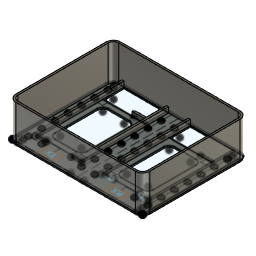
Pluto_Case_V2.8_lite (Autodesk Fusion 360 design; units mm, degrees)
Autodesk Fusion 360 part; units mm, degrees
sketch "base" plane through (0, 0, 0) normal (0, 0, 1) x (1, 0, 0)
  line L0 (10, 0) -> (235, 0)
  line L1 (245, 10) -> (245, 180)
  line L2 (235, 190) -> (10, 190)
  line L3 (0, 180) -> (0, 10)
  line L4 (0, 0) -> (10, 0) construction
  line L5 (0, 190) -> (10, 190) construction
  line L6 (10, 190) -> (10, 170) construction
  circle A0 centre (10, 170) radius 5
  line L7 (10, 170) -> (10, 145) construction
  line L8 (10, 145) -> (10, 120) construction
  line L9 (10, 120) -> (10, 95) construction
  line L10 (10, 95) -> (10, 70) construction
  line L11 (10, 70) -> (10, 45) construction
  line L12 (10, 45) -> (10, 20) construction
  circle A1 centre (10, 145) radius 5
  circle A2 centre (10, 120) radius 5
  circle A3 centre (10, 95) radius 5
  circle A4 centre (10, 70) radius 5
  circle A5 centre (10, 45) radius 5
  circle A6 centre (10, 20) radius 5
  line L13 (0, 190) -> (20, 190) construction
  line L14 (20, 190) -> (100, 190) construction
  line L15 (20, 190) -> (100, 190)
  line L16 (100, 190) -> (100, 150)
  line L17 (100, 150) -> (20, 150)
  line L18 (20, 160) -> (20, 190)
  line L19 (30, 150) -> (100, 150)
  line L20 (100, 150) -> (100, 30)
  line L21 (100, 30) -> (20, 30)
  line L22 (20, 30) -> (20, 150)
  line L23 (20, 150) -> (30, 150) construction
  line L24 (30, 150) -> (30, 140) construction
  line L25 (30, 140) -> (20, 140) construction
  line L26 (20, 140) -> (20, 150) construction
  line L27 (100, 30) -> (90, 30) construction
  line L28 (90, 30) -> (90, 40) construction
  line L29 (90, 40) -> (100, 40) construction
  line L30 (100, 40) -> (100, 30) construction
  line L31 (40, 140) -> (80, 140)
  line L32 (90, 130) -> (90, 50)
  line L33 (80, 40) -> (40, 40)
  line L34 (30, 50) -> (30, 130)
  line L35 (20, 190) -> (16, 190) construction
  line L36 (100, 190) -> (104, 190) construction
  line L37 (16, 190) -> (16, 30)
  line L38 (20, 26) -> (33, 26)
  line L39 (36, 29) -> (36, 30)
  line L40 (104, 190) -> (104, 30)
  line L41 (100, 26) -> (87, 26)
  line L42 (84, 29) -> (84, 30)
  line L43 (100, 190) -> (110, 190) construction
  line L44 (0, 0) -> (100, 0) construction
  line L45 (100, 0) -> (110, 0) construction
  line L46 (110, 190) -> (110, 170) construction
  line L47 (110, 170) -> (110, 145) construction
  line L48 (110, 145) -> (110, 120) construction
  line L49 (110, 120) -> (110, 95) construction
  line L50 (110, 95) -> (110, 70) construction
  line L51 (110, 70) -> (110, 45) construction
  line L52 (110, 45) -> (110, 20) construction
  circle A7 centre (110, 170) radius 5
  circle A8 centre (110, 145) radius 5
  circle A9 centre (110, 120) radius 5
  circle A10 centre (110, 95) radius 5
  circle A11 centre (110, 70) radius 5
  circle A12 centre (110, 45) radius 5
  circle A13 centre (110, 20) radius 5
  line L53 (0, 190) -> (122.5, 190) construction
  line L54 (0, 0) -> (122.5, 0) construction
  line L55 (122.5, 190) -> (122.5, 0) construction
  line L56 (10, 20) -> (35, 20) construction
  circle A14 centre (35, 20) radius 5
  arc A15 (40, 140) -> (30, 130) centre (40, 130) ccw
  arc A16 (90, 130) -> (80, 140) centre (80, 130) ccw
  arc A17 (80, 40) -> (90, 50) centre (80, 50) ccw
  arc A18 (30, 50) -> (40, 40) centre (40, 50) ccw
  arc A19 (16, 30) -> (20, 26) centre (20, 30) ccw
  arc A20 (100, 26) -> (104, 30) centre (100, 30) ccw
  circle A21 centre (135, 70) radius 5
  line L57 (155, 40) -> (145, 40) construction
  line L58 (235, 190) -> (235, 170) construction
  arc A22 (141, 30) -> (145, 26) centre (145, 30) ccw
  line L59 (141, 190) -> (141, 30)
  line L60 (145, 0) -> (135, 0) construction
  line L61 (145, 26) -> (158, 26)
  line L62 (145, 150) -> (145, 30)
  line L63 (225, 150) -> (215, 150) construction
  line L64 (225, 190) -> (229, 190) construction
  arc A23 (155, 50) -> (165, 40) centre (165, 50) ccw
  line L65 (209, 29) -> (209, 30)
  circle A24 centre (135, 45) radius 5
  line L66 (161, 29) -> (161, 30)
  line L67 (135, 45) -> (135, 20) construction
  circle A25 centre (135, 20) radius 5
  line L68 (245, 190) -> (225, 190) construction
  line L69 (245, 190) -> (235, 190) construction
  line L70 (155, 30) -> (155, 40) construction
  line L71 (235, 170) -> (235, 145) construction
  line L72 (145, 30) -> (155, 30) construction
  line L73 (145, 40) -> (145, 30) construction
  circle A26 centre (235, 170) radius 5
  line L74 (135, 70) -> (135, 45) construction
  line L75 (215, 150) -> (215, 140) construction
  line L76 (225, 190) -> (145, 190) construction
  circle A27 centre (235, 20) radius 5
  circle A28 centre (235, 145) radius 5
  arc A29 (225, 26) -> (229, 30) centre (225, 30) ccw
  arc A30 (205, 40) -> (215, 50) centre (205, 50) ccw
  circle A31 centre (235, 70) radius 5
  circle A32 centre (235, 120) radius 5
  line L77 (225, 150) -> (225, 190)
  circle A33 centre (210, 20) radius 5
  arc A34 (215, 130) -> (205, 140) centre (205, 130) ccw
  line L78 (215, 140) -> (225, 140) construction
  line L79 (235, 45) -> (235, 20) construction
  circle A35 centre (235, 45) radius 5
  line L80 (225, 140) -> (225, 150) construction
  line L81 (235, 145) -> (235, 120) construction
  line L82 (235, 120) -> (235, 95) construction
  line L83 (235, 20) -> (210, 20) construction
  line L84 (225, 26) -> (212, 26)
  line L85 (229, 190) -> (229, 30)
  line L86 (225, 30) -> (225, 150)
  line L87 (235, 70) -> (235, 45) construction
  line L88 (215, 50) -> (215, 130)
  circle A36 centre (235, 95) radius 5
  line L89 (235, 95) -> (235, 70) construction
  line L90 (205, 140) -> (165, 140)
  circle A37 centre (135, 95) radius 5
  line L91 (135, 190) -> (135, 170) construction
  line L92 (145, 190) -> (141, 190) construction
  line L93 (145, 30) -> (225, 30)
  line L94 (135, 120) -> (135, 95) construction
  line L95 (135, 145) -> (135, 120) construction
  circle A38 centre (135, 120) radius 5
  circle A39 centre (135, 145) radius 5
  circle A40 centre (135, 170) radius 5
  line L96 (145, 150) -> (225, 150)
  line L97 (225, 190) -> (145, 190)
  arc A41 (165, 140) -> (155, 130) centre (165, 130) ccw
  line L98 (225, 150) -> (155, 150)
  line L99 (135, 170) -> (135, 145) construction
  line L100 (145, 190) -> (145, 160)
  line L101 (245, 0) -> (145, 0) construction
  line L102 (135, 95) -> (135, 70) construction
  line L103 (245, 0) -> (235, 0) construction
  line L104 (155, 130) -> (155, 50)
  line L105 (145, 190) -> (135, 190) construction
  line L106 (165, 40) -> (205, 40)
  line L107 (100, 150) -> (75, 150)
  line L108 (79, 154) -> (100, 154)
  line L109 (100, 154) -> (100, 150)
  arc A42 (79, 154) -> (75, 150) centre (79, 150) ccw
  line L110 (225, 150) -> (200, 150)
  line L111 (204, 154) -> (225, 154)
  line L112 (225, 154) -> (225, 150)
  arc A43 (204, 154) -> (200, 150) centre (204, 150) ccw
  arc A44 (10, 190) -> (0, 180) centre (10, 180) ccw
  arc A45 (0, 10) -> (10, 0) centre (10, 10) ccw
  arc A46 (235, 0) -> (245, 10) centre (235, 10) ccw
  arc A47 (245, 180) -> (235, 190) centre (235, 180) ccw
  line L113 (235, 193.6) -> (10, 193.6)
  arc A48 (10, 193.6) -> (-3.6, 180) centre (10, 180) ccw
  line L114 (-3.6, 180) -> (-3.6, 10)
  arc A49 (-3.6, 10) -> (10, -3.6) centre (10, 10) ccw
  line L115 (10, -3.6) -> (235, -3.6)
  arc A50 (235, -3.6) -> (248.6, 10) centre (235, 10) ccw
  line L116 (248.6, 10) -> (248.6, 180)
  arc A51 (248.6, 180) -> (235, 193.6) centre (235, 180) ccw
  arc A52 (33, 26) -> (36, 29) centre (33, 29) ccw
  arc A53 (84, 29) -> (87, 26) centre (87, 29) ccw
  arc A54 (158, 26) -> (161, 29) centre (158, 29) ccw
  arc A55 (209, 29) -> (212, 26) centre (212, 29) ccw
  arc A56 (20, 160) -> (30, 150) centre (30, 160) ccw
  arc A57 (145, 160) -> (155, 150) centre (155, 160) ccw
  line L117 (20, 150) -> (20, 160)
  line L118 (145, 150) -> (145, 160)
  line L119 (245, 190) -> (245, 189.2174)
  line L120 (245, 180) -> (245, 10)
  line L121 (245, 0.7826) -> (245, 0)
  line L122 (45, 5) -> (75, 5) construction
  line L123 (75, 5) -> (75, 20) construction
  line L124 (75, 20) -> (45, 20) construction
  line L125 (45, 20) -> (45, 5) construction
  line L126 (20, 30) -> (60, 30) construction
  line L127 (60, 30) -> (60, 20) construction
  line L128 (225, 30) -> (185, 30) construction
  line L129 (185, 30) -> (185, 20) construction
  line L130 (170, 5) -> (200, 5) construction
  line L131 (200, 5) -> (200, 20) construction
  line L132 (200, 20) -> (170, 20) construction
  line L133 (170, 20) -> (170, 5) construction
  point P0 (245, 0)
  point P1 (16, 26)
  point P2 (36, 26)
  point P3 (104, 26)
  point P4 (84, 26)
  point P5 (245, 0)
  point P6 (229, 26)
  point P7 (141, 26)
  point P8 (245, 0)
  dimension "d4" = 245
  dimension "d5" = 190
  dimension "d15" = 10
  dimension "d16" = 10
  dimension "d17" = 20
  dimension "d18" = 10
  dimension "d19" = 25
  dimension "d20" = 25
  dimension "d21" = 25
  dimension "d22" = 25
  dimension "d23" = 25
  dimension "d24" = 25
  dimension "d25" = 10
  dimension "d26" = 10
  dimension "d27" = 10
  dimension "d28" = 10
  dimension "d29" = 10
  dimension "d30" = 10
  dimension "d31" = 20
  dimension "d32" = 80
  dimension "d33" = 80
  dimension "d34" = 40
  dimension "d35" = 80
  dimension "d36" = 120
  dimension "d37" = 10
  dimension "d38" = 10
  dimension "d39" = 10
  dimension "d40" = 10
  dimension "d41" = 4
  dimension "d42" = 4
  dimension "d43" = 164
  dimension "d44" = 20
  dimension "d45" = 4
  dimension "d46" = 164
  dimension "d47" = 20
  dimension "d48" = 10
  dimension "d49" = 100
  dimension "d50" = 10
  dimension "d51" = 20
  dimension "d52" = 25
  dimension "d53" = 25
  dimension "d54" = 25
  dimension "d55" = 25
  dimension "d56" = 25
  dimension "d57" = 25
  dimension "d58" = 10
  dimension "d59" = 10
  dimension "d60" = 10
  dimension "d61" = 10
  dimension "d62" = 10
  dimension "d63" = 10
  dimension "d64" = 10
  dimension "d65" = 122.5
  dimension "d66" = 122.5
  dimension "d67" = 25
  dimension "d68" = 10
  dimension "d69" = 10
  dimension "d70" = 10
  dimension "d71" = 10
  dimension "d72" = 10
  dimension "d73" = 4
  dimension "d74" = 4
  dimension "d75" = 25
  dimension "d76" = 4
  dimension "d77" = 4
  dimension "d78" = 25
  dimension "d79" = 4
  dimension "d80" = 4
  dimension "d81" = 3.6
  dimension "d82" = 10
  dimension "d83" = 10
  dimension "d84" = 10
  dimension "d85" = 10
  dimension "d92" = 3
  dimension "d93" = 3
  dimension "d94" = 3
  dimension "d95" = 3
  dimension "d96" = 10
  dimension "d97" = 10
  dimension "d104" = 10
  dimension "d105" = 10
  dimension "d106" = 10
  dimension "d107" = 10
  dimension "d108" = 15
  dimension "d109" = 30
  dimension "d110" = 30
  dimension "d111" = 15
  text T0 "TX" font "Arial" height 10 align centre middle in box 30 x 15 at (45, 5) x (1, 0) y (0, 1) spacing 1 kerned mirrored across mirrored up
  text T1 "RX" font "Arial" height 10 align centre middle in box 30 x 15 at (170, 5) x (1, 0) y (0, 1) spacing 1 kerned mirrored across mirrored up
  constraint horizontal L0
  constraint vertical L1
  constraint horizontal L2
  constraint vertical L3
  constraint coincident L4.start L44.start
  constraint perpendicular L3 L4
  constraint coincident L2 L5.end
  constraint vertical L6
  constraint coincident L6.end A0.centre
  constraint parallel L6 L7
  constraint parallel L7 L8
  constraint parallel L8 L9
  constraint parallel L9 L10
  constraint parallel L10 L11
  constraint parallel L11 L12
  constraint coincident L7.end L8.start
  constraint coincident L8.end L9.start
  constraint coincident L9.end L10.start
  constraint coincident L10.end L11.start
  constraint coincident L11.end L12.start
  constraint coincident L12.end A6.centre
  constraint horizontal L13
  constraint horizontal L14
  constraint horizontal L15
  constraint vertical L16
  constraint horizontal L17
  constraint vertical L18
  constraint horizontal L19
  constraint vertical L20
  constraint horizontal L21
  constraint vertical L22
  constraint horizontal L23
  constraint vertical L24
  constraint horizontal L25
  constraint vertical L26
  constraint horizontal L27
  constraint vertical L28
  constraint horizontal L29
  constraint vertical L30
  constraint horizontal L31
  constraint vertical L32
  constraint horizontal L33
  constraint vertical L34
  constraint perpendicular L18 L35
  constraint perpendicular L16 L36
  constraint perpendicular L35 L37
  constraint perpendicular L37 L38
  constraint perpendicular L21 L39
  constraint perpendicular L36 L40
  constraint perpendicular L40 L41
  constraint coincident L21 L42.end
  constraint perpendicular L21 L42
  constraint perpendicular L40 L43
  constraint perpendicular L3 L44
  constraint perpendicular L32 L45
  constraint perpendicular L43 L46
  constraint parallel L46 L47
  constraint parallel L40 L48
  constraint parallel L48 L49
  constraint parallel L49 L50
  constraint perpendicular L29 L51
  constraint parallel L51 L52
  constraint coincident L46.end L47.start
  constraint coincident L47.end L48.start
  constraint coincident L48.end L49.start
  constraint coincident L49.end L50.start
  constraint coincident L50.end L51.start
  constraint coincident L51.end L52.start
  constraint coincident L52.end A13.centre
  constraint perpendicular L3 L53
  constraint parallel L0 L54
  constraint perpendicular L12 L56
  constraint coincident L56.end A14.centre
  constraint coincident L24.end L31
  constraint coincident L24.end L34
  constraint tangent L31 A15
  constraint tangent L34 A15
  constraint tangent L31 A16
  constraint tangent L32 A16
  constraint coincident L28.end L33
  constraint coincident L28.end L32
  constraint tangent L33 A17
  constraint tangent L32 A17
  constraint tangent L33 A18
  constraint tangent L34 A18
  constraint coincident P1 L37
  constraint coincident P1 L38
  constraint tangent L37 A19
  constraint tangent L38 A19
  constraint coincident P3 L40
  constraint coincident P3 L41
  constraint tangent L40 A20
  constraint tangent L41 A20
  constraint symmetric L4.start L55 P8
  constraint symmetric L5.start L55 L68.start
  constraint symmetric L0.start L55 L0.end
  constraint symmetric L2.end L55 L2.start
  constraint symmetric L6.end L55 L58.end
  constraint symmetric A0 L55 A26
  constraint symmetric L7.end L55 L71.end
  constraint symmetric L8.end L55 A32.centre
  constraint symmetric L9.end L55 L82.end
  constraint symmetric L10.end L55 A31.centre
  constraint symmetric L11.end L55 L79.start
  constraint symmetric L12.end L55 A27.centre
  constraint symmetric A1 L55 A28
  constraint symmetric A2 L55 A32
  constraint symmetric A3 L55 A36
  constraint symmetric A4 L55 A31
  constraint symmetric A5 L55 A35
  constraint symmetric A6 L55 A27
  constraint symmetric L13.end L55 L64.start
  constraint symmetric L14.end L55 L76.end
  constraint symmetric L16.end L55 L62.start
  constraint symmetric L17.end L55 L63.start
  constraint symmetric L20.end L55 A22.centre
  constraint symmetric L21.end L55 A29.centre
  constraint symmetric L19.start L55 L63.end
  constraint symmetric L24.end L55 L75.end
  constraint symmetric L25.end L55 L78.end
  constraint symmetric L27.end L55 L70.start
  constraint symmetric L28.end L55 L57.start
  constraint symmetric L29.end L55 L57.end
  constraint symmetric L35.end L55 L64.end
  constraint symmetric L36.end L55 L59.start
  constraint symmetric P1 L55 P6
  constraint symmetric L39.end L55 L65.end
  constraint symmetric P3 L55 P7
  constraint symmetric L42.end L55 L66.end
  constraint symmetric L43.end L55 L91.start
  constraint symmetric L44.end L55 L60.start
  constraint symmetric L45.end L55 L60.end
  constraint symmetric L46.end L55 L91.end
  constraint symmetric L47.end L55 L95.start
  constraint symmetric L48.end L55 L94.start
  constraint symmetric L49.end L55 A37.centre
  constraint symmetric L50.end L55 A21.centre
  constraint symmetric L51.end L55 A24.centre
  constraint symmetric L52.end L55 L67.end
  constraint symmetric A7 L55 A40
  constraint symmetric A8 L55 A39
  constraint symmetric A9 L55 A38
  constraint symmetric A10 L55 A37
  constraint symmetric A11 L55 A21
  constraint symmetric A12 L55 A24
  constraint symmetric A13 L55 A25
  constraint symmetric L55 L12.end A27.centre
  constraint symmetric L55 L56.end A33.centre
  constraint symmetric L55 A14 A33
  constraint symmetric L55 L31.start A34.end
  constraint symmetric L55 L34.end A34.start
  constraint symmetric L55 A15 A34
  constraint symmetric L55 L31.end L90.end
  constraint symmetric L55 L32.start A41.end
  constraint symmetric L55 A16 A41
  constraint symmetric L55 L33.start A23.end
  constraint symmetric L55 L32.end A23.start
  constraint symmetric L55 A17 A23
  constraint symmetric L55 L33.end A30.start
  constraint symmetric L55 L34.start A30.end
  constraint symmetric L55 A18 A30
  constraint symmetric L55 L37.end A29.end
  constraint symmetric L55 L38.start A29.start
  constraint symmetric L55 A19 A29
  constraint symmetric L55 L40.end A22.start
  constraint symmetric L55 L41.start A22.end
  constraint symmetric L55 A20 A22
  constraint horizontal L107
  constraint horizontal L108
  constraint vertical L109
  constraint tangent L108 A42
  constraint coincident L107.end A42.end
  constraint horizontal L110
  constraint horizontal L111
  constraint vertical L112
  constraint tangent L111 A43
  constraint coincident L110.end A43.end
  constraint coincident L5.start L3
  constraint coincident L5.start L2
  constraint tangent L3 A44
  constraint tangent L2 A44
  constraint coincident L4.start L0
  constraint coincident L4.start L3
  constraint tangent L0 A45
  constraint tangent L3 A45
  constraint coincident P8 L0
  constraint coincident P8 L1
  constraint tangent L0 A46
  constraint tangent L1 A46
  constraint tangent L1 A47
  constraint tangent L2 A47
  constraint coincident P2 L38
  constraint coincident P2 L39
  constraint tangent L38 A52
  constraint tangent L39 A52
  constraint coincident P4 L41
  constraint coincident P4 L42
  constraint tangent L41 A53
  constraint tangent L42 A53
  constraint tangent L61 A54
  constraint tangent L66 A54
  constraint tangent L65 A55
  constraint tangent L84 A55
  constraint coincident L17.end L19
  constraint coincident L17.end L18
  constraint tangent L19 A56
  constraint tangent L18 A56
  constraint coincident L62.start L98
  constraint coincident L62.start L100
  constraint tangent L98 A57
  constraint tangent L100 A57
  constraint coincident A51 L119.end
  constraint collinear L119 L120
  constraint coincident A50 L121.start
  constraint collinear L120 L121
  constraint midpoint L21 L126.end
  constraint perpendicular L126 L127
  constraint coincident L127.end
  constraint midpoint L93 L128.end
  constraint perpendicular L128 L129
  constraint coincident L129.end
  measures "d4" distance of L4.start P8
  measures "d5" distance of L4.start L5.start
  measures "d15" distance of L4.start L0.start
  measures "d16" distance of L5.start L2.end
  measures "d17" distance of L2.end L6.end
  measures "d18" diameter of A0
  measures "d19" distance of L6.end L7.end
  measures "d20" distance of L7.end L8.end
  measures "d21" distance of L8.end L9.end
  measures "d22" distance of L9.end L10.end
  measures "d23" distance of L10.end L11.end
  measures "d24" distance of L11.end L12.end
  measures "d25" diameter of A1
  measures "d26" diameter of A2
  measures "d27" diameter of A3
  measures "d28" diameter of A4
  measures "d29" diameter of A5
  measures "d30" diameter of A6
  measures "d31" distance of L5.start L13.end
  measures "d32" distance of L13.end L14.end
  measures "d33" distance of L13.end L14.end
  measures "d34" distance of L13.end L17.end
  measures "d35" distance of L17.end L16.end
  measures "d36" distance of L17.end L21.end
  measures "d37" distance of L17.end L19.start
  measures "d38" distance of L17.end L25.end
  measures "d39" distance of L20.end L27.end
  measures "d40" distance of L20.end L29.end
  measures "d41" distance of L13.end L35.end
  measures "d42" distance of L14.end L36.end
  measures "d43" distance of L35.end P1
  measures "d44" distance of P1 P2
  measures "d45" distance of P2 L39.end
  measures "d46" distance of L36.end P3
  measures "d47" distance of P3 P4
  measures "d48" distance of L14.end L43.end
  measures "d49" distance of L4.start L44.end
  measures "d50" distance of L44.end L45.end
  measures "d51" distance of L43.end L46.end
  measures "d52" distance of L46.end L47.end
  measures "d53" distance of L47.end L48.end
  measures "d54" distance of L48.end L49.end
  measures "d55" distance of L49.end L50.end
  measures "d56" distance of L50.end L51.end
  measures "d57" distance of L51.end L52.end
  measures "d58" diameter of A7
  measures "d59" diameter of A8
  measures "d60" diameter of A9
  measures "d61" diameter of A10
  measures "d62" diameter of A11
  measures "d63" diameter of A12
  measures "d64" diameter of A13
  measures "d65" distance of L5.start L53.end
  measures "d66" distance of L4.start L54.end
  measures "d67" distance of L12.end L56.end
  measures "d68" diameter of A14
  measures "d69" radius of A15
  measures "d70" radius of A16
  measures "d71" radius of A17
  measures "d72" radius of A18
  measures "d73" radius of A19
  measures "d74" radius of A20
  measures "d75" distance of L16.end L107.end
  measures "d76" distance of L16.end L108.end
  measures "d77" radius of A42
  measures "d78" distance of L63.start L110.end
  measures "d79" distance of L63.start L111.end
  measures "d80" radius of A43
  measures "d82" radius of A44
  measures "d83" radius of A45
  measures "d84" radius of A46
  measures "d85" radius of A47
  measures "d92" radius of A52
  measures "d93" radius of A53
  measures "d94" radius of A54
  measures "d95" radius of A55
  measures "d96" radius of A56
  measures "d97" radius of A57
  measures "d105" distance of L126.end L127.end
  measures "d106" distance of L128.end L129.end
extrude "Extrude2" add sketch "base" along normal blind 8 contours L77 L96 L98 L110 L111 L112 A43 | L16 L17 L19 L107 L108 L109 A42 makes body 1 at (91.6667, 150, 5.3333) makes body 2 at (208.3333, 150, 5.3333)
extrude "Extrude4" add sketch "base" against normal blind 2.8 separate body contours L0 L1 L2 L3 L21 L37 L38 L39 L40 L41 L42 A19 A20 A22 L59 L61 L65 L66 A29 L84 L85 L93 A44 A45 A46 A47 A52 A53 A54 A55 L120 | L2 L18 L21 L22 L37 L38 L39 A19 A52 L117 | L2 L65 A29 L77 L84 L85 L86 L93 L112 A55 | L2 L16 L20 L21 L40 L41 L42 A20 L109 A53 | L17 A56 L117 | L2 A22 L59 L61 L62 L66 L93 L100 A54 L118 | L77 L96 L98 L110 L111 L112 A43 | L16 L17 L19 L107 L108 L109 A42 | L17 L19 L20 L21 L22 L107 | L96 A57 L118 | L62 L86 L93 L96 L98 L110 | L113 A48 L114 A49 L115 A50 L116 A51 makes body 3
extrude "Extrude5" add sketch "base" along normal blind 10 contours L2 L18 L21 L22 L37 L38 L39 A19 A52 L117 | L2 L65 A29 L77 L84 L85 L86 L93 L112 A55 | L2 L16 L20 L21 L40 L41 L42 A20 L109 A53 | L2 A22 L59 L61 L62 L66 L93 L100 A54 L118 bodies 1 2 3
extrude "Extrude6" add sketch "base" along normal blind 67 separate body contours L113 A48 L114 A49 L115 A50 L116 A51 makes body 4
extrude "Extrude7" cut sketch "base" against normal blind 1 text T0 T1 bodies 1
combine "Combine1" operation add target body 1 tool bodies 4
copy_body "Body->Comp1" bodies 1 removing the originals makes body 5 in component "case"
component "case" placed x (1, 0, 0) y (0, 1, 0) z (0, 0, 1) at (0, 0, 0)
equation "inner_base_length = 245 mm"
equation "inner_base_width = 190 mm"
equation "wall_height = 67 mm"
equation "d4 = inner_base_length"
equation "d5 = inner_base_width"
equation "wall_thickness = 3.6 mm"
equation "lock_thickness = 4 mm"
equation "lock_height = 10 mm"
equation "lock_side_length = 40 mm"
equation "lock_top_length = 15 mm"
equation "hole_diameter = 10 mm"
equation "pluto_width = 80 mm"
equation "pluto_length = 120 mm"
equation "base_thickness = 2.8 mm"
equation "d18 = hole_diameter"
equation "d25 = hole_diameter"
equation "d26 = hole_diameter"
equation "d27 = hole_diameter"
equation "d28 = hole_diameter"
equation "d29 = hole_diameter"
equation "d30 = hole_diameter"
equation "d32 = pluto_width"
equation "d33 = pluto_width"
equation "d35 = pluto_width"
equation "d36 = pluto_length"
equation "d58 = hole_diameter"
equation "d59 = hole_diameter"
equation "d60 = hole_diameter"
equation "d61 = hole_diameter"
equation "d62 = hole_diameter"
equation "d63 = hole_diameter"
equation "d64 = hole_diameter"
equation "d65 = inner_base_length / 2"
equation "d66 = inner_base_length / 2"
equation "d68 = hole_diameter"
equation "d81 = wall_thickness"
equation "d98 = -base_thickness"
equation "d102 = wall_height"
